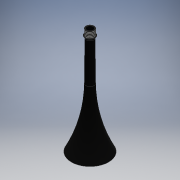
# Autodesk Inventor part: Horn_B
Saved by Autodesk Inventor 2016 (Build 200138000, 138)
## iProperties
Created: 2016-05-21
Part Number: Horn_B
Material: Steel, Cast
Document SubType Name: Modeling
Designer: agmle
Density: 7.85 g/cm^3
Appearance: Glossy - Black
Mass: 352.907 g
Surface Area: 586.282 cm^2
Volume: 44.9563 cm^3
Author: agmle
Autodesk Inventor part; units mm, degrees
ref_plane "YZ Plane" through (0, 0, 0) normal (1, 0, 0) x (0, 1, 0)
ref_plane "XZ Plane" through (0, 0, 0) normal (0, 1, 0) x (-1, 0, 0)
ref_plane "XY Plane" through (0, 0, 0) normal (0, 0, 1) x (1, 0, 0)
sketch "Sketch1" plane through (0, 0, 0) normal (0, 1, 0) x (-1, 0, 0)
  line L0 (0, 0) -> (0, -270.8) construction
  line L1 (0, -270.8) -> (47.15, -270.8) construction
  line L2 (0, -120.8) -> (10.5, -120.8) construction
  line L3 (0, -20.8) -> (9.5, -20.8) construction
  line L4 (0, -15.3) -> (12.6, -15.3) construction
  line L5 (0, 0) -> (10.5, 0) construction
  line L6 (10.5, 0) -> (10.5, -15.3)
  line L7 (10.5, -15.3) -> (12.6, -15.3)
  line L8 (12.6, -15.3) -> (9.5, -20.8)
  line L9 (10.5, -120.8) -> (9.5, -20.8)
  arc A0 (10.5, -120.8) -> (47.15, -270.8) centre (349.6639, -117.4084) ccw
  arc A1 (8.9999, -120.8) -> (45.4691, -270.8) centre (349.6639, -117.4084) ccw
  line L10 (8.9999, -120.8) -> (7.7919, 0)
  line L11 (10.5, 0) -> (7.7919, 0)
  arc A2 (45.4691, -270.8) -> (47.15, -270.8) centre (46.3096, -270.3762) ccw
  dimension "d0" = 15.3
  dimension "d1" = 5.5
  dimension "d2" = 100
  dimension "d3" = 150
  dimension "d4" = 47.15
  dimension "d5" = 10.5
  dimension "d6" = 9.5
  dimension "d7" = 12.6
  dimension "d8" = 10.5
  dimension "d9" = 1.5
  constraints: 24 end point, 7 point on line, 6 point on circle, 4 horizontal, 3 centre point, 2 tangent, 2 vertical, 1 collinear, 1 concentric, 1 parallel, 1 perpendicular
  measures "d0" distance between parallel lines of L4 L5
  measures "d1" distance between parallel lines of L3 L4
  measures "d2" distance between parallel lines of L2 L3
  measures "d3" distance between parallel lines of L1 L2
  measures "d4" distance of L0.end L1.end
  measures "d5" distance of L2.start L2.end
  measures "d6" distance of L3.start L3.end
  measures "d7" distance of L4.start L4.end
  measures "d8" distance of L0.start L5.end
  measures "d9" distance between parallel lines of L10 L9
revolve "Revolution1" add sketch "Sketch1" angle 360 about axis through (0, 0, 0) along (0, 0, -1)
thread "Thread1" size "M22x3" class "6g" standard "ANSI Metric M Profile" full length
equation "\"d0\" = Mount_Length"
equation "\"d1\" = Mount_Flange_Length"
equation "\"d2\" = Transition_Length"
equation "\"d3\" = Flare_Length"
equation "\"d4\" = Flare_Diameter"
equation "\"d5\" = Transition_Diameter"
equation "\"d6\" = Tail_Diameter"
equation "\"d7\" = Mount_Flange_Diameter"
equation "\"d8\" = Mount_Diameter"
equation "\"d9\" = Bell_Thickness"
equation "\"Transition_Length\" = 100"
equation "\"Mount_Length\" = 15.3"
equation "\"Mount_Flange_Length\" = 5.5"
equation "\"Flare_Length\" = 150"
equation "\"Flare_Diameter\" = 47.15"
equation "\"Transition_Diameter\" = 10.5"
equation "\"Tail_Diameter\" = 9.5"
equation "\"Mount_Flange_Diameter\" = 12.6"
equation "\"Mount_Diameter\" = 10.5"
equation "\"Bell_Thickness\" = 1.5"
body "Solid1"
